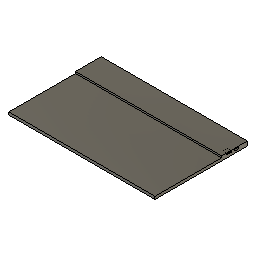
Monitor_v1 (Autodesk Fusion 360 design; units mm, degrees)
Autodesk Fusion 360 part; units mm, degrees
note: some values were not read from the file. Set by a fixed rule: which sketch regions a step uses.
sketch "Sketch1" plane through (0, 0, 0) normal (0, 0, 1) x (1, 0, 0)
  line L0 (0, 0) -> (364, 0)
  line L1 (364, 0) -> (364, -230)
  line L2 (364, -230) -> (0, -230)
  line L3 (0, -230) -> (0, 0)
  line L4 (364, -64) -> (0, -64)
  constraint horizontal L0
  constraint vertical L1
  constraint horizontal L2
  constraint vertical L3
  constraint coincident L0.start L3.end
  constraint coincident L1 L4.start
  constraint coincident L3 L4.end
  constraint perpendicular L3 L4
extrude "Extrude1" add sketch "Sketch1" along normal blind 6.85 contours L1 L2 L3 L4
extrude "Extrude2" add sketch "Sketch1" along normal blind 11.1 contours L0 L1 L3 L4
sketch "Sketch2" plane through (0, 0, 0) normal (-1, 0, 0) x (0, -1, 0)
  line L0 (0, 0) -> (230, 0)
  line L1 (230, 0) -> (230, 6.85)
  line L2 (230, 6.85) -> (64, 6.85)
  line L3 (64, 6.85) -> (64, 11.1)
  line L4 (64, 11.1) -> (0, 11.1)
  line L5 (0, 11.1) -> (0, 0)
  circle A0 centre (45, 8.1) radius 2
  line L6 (36, 8.5) -> (26, 8.5)
  line L7 (26, 8.5) -> (26, 5.9)
  line L8 (26, 5.9) -> (36, 5.9)
  line L9 (36, 5.9) -> (36, 8.5)
  line L10 (21.4, 9.1) -> (11.4, 9.1)
  line L11 (11.4, 9.1) -> (11.4, 5.45)
  line L12 (11.4, 5.45) -> (21.4, 5.45)
  line L13 (21.4, 5.45) -> (21.4, 9.1)
  dimension "d10" = 4
  constraint horizontal L6
  constraint vertical L7
  constraint horizontal L8
  constraint vertical L9
  constraint horizontal L10
  constraint vertical L11
  constraint horizontal L12
  constraint vertical L13
  measures "d10" diameter of A0
extrude "Extrude3" add sketch "Sketch2" along normal blind 0.5 contours A0
extrude "Extrude4" cut sketch "Sketch2" against normal blind 9 contours L6 L7 L8 L9 | L10 L11 L12 L13
sketch "Sketch3" plane through (0, 0, 5.9) normal (0, 0, 1) x (-1, 0, 0)
  line L0 (0, 26) -> (0, 36)
  line L1 (0, 36) -> (-9, 36)
  line L2 (-9, 36) -> (-9, 26)
  line L3 (-9, 26) -> (0, 26)
  circle A0 centre (-4, 31) radius 4.5
extrude "Extrude5" add sketch "Sketch3" along normal blind 2.6 contours L0 A0 | L0 A0
sketch "Sketch4" plane through (364, 0, 0) normal (1, 0, 0) x (0, 1, 0)
  line L0 (-230, 0) -> (0, 0)
  line L1 (0, 0) -> (0, 11.1)
  line L2 (0, 11.1) -> (-64, 11.1)
  line L3 (-64, 11.1) -> (-64, 6.85)
  line L4 (-64, 6.85) -> (-230, 6.85)
  line L5 (-230, 6.85) -> (-230, 0)
  line L6 (-21, 8.8) -> (-31, 8.8)
  line L7 (-31, 8.8) -> (-31, 5.15)
  line L8 (-31, 5.15) -> (-21, 5.15)
  line L9 (-21, 5.15) -> (-21, 8.8)
  line L10 (-39.5, 9.4) -> (-51, 9.4)
  line L11 (-51, 9.4) -> (-51, 6.9)
  line L12 (-51, 6.9) -> (-39.5, 6.9)
  line L13 (-39.5, 6.9) -> (-39.5, 9.4)
  constraint horizontal L6
  constraint vertical L7
  constraint horizontal L8
  constraint vertical L9
  constraint horizontal L10
  constraint vertical L11
  constraint horizontal L12
  constraint vertical L13
extrude "Extrude6" cut sketch "Sketch4" against normal blind 10 contours L6 L7 L8 L9 | L10 L11 L12 L13
